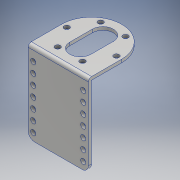
# Autodesk Inventor part: bepf_podwozie_lacznik_silnika
Saved by Autodesk Inventor 2017 (Build 210142000, 142)
## iProperties
Created: 2016-11-23
Part Number: bepf_podwozie_lacznik_silnika
Material: Aluminium 6061
Document SubType Name: Modeling
Designer: gagato
Density: 2.7 g/cm^3
Appearance: Aluminium — płaski
Mass: 14.4645 g
Surface Area: 63.668 cm^2
Volume: 5.35723 cm^3
Author: gagato
Autodesk Inventor part; units mm, degrees
ref_plane "YZ Plane" through (0, 0, 0) normal (1, 0, 0) x (0, 1, 0)
ref_plane "XZ Plane" through (0, 0, 0) normal (0, 1, 0) x (-1, 0, 0)
ref_plane "XY Plane" through (0, 0, 0) normal (0, 0, 1) x (1, 0, 0)
sketch "Szkic5" plane through (0, 0, 0) normal (0, 0, 1) x (1, 0, 0)
  line L0 (-18.8, 0) -> (18.8, 0)
  line L1 (0, 0) -> (0, 20.8) construction
  arc A0 (18.8, 20.8) -> (-18.8, 20.8) centre (0, 20.8) ccw
  line L2 (-18.8, 0) -> (-18.8, 20.8)
  line L3 (18.8, 0) -> (18.8, 20.8)
  circle A1 centre (0, 20.8) radius 15.5 construction
  line L4 (0, 27.8) -> (0, 13.8) construction
  line L5 (0, 27.8) -> (0, 13.8) construction
  line L6 (-6.6, 27.8) -> (-6.6, 13.8)
  line L7 (6.6, 13.8) -> (6.6, 27.8)
  arc A2 (6.6, 27.8) -> (-6.6, 27.8) centre (0, 27.8) ccw
  arc A3 (-6.6, 13.8) -> (6.6, 13.8) centre (0, 13.8) ccw
  point P0 (-15.5, 20.8)
  point P1 (0, 20.8)
  dimension "d35" = 31
  dimension "d26" = 37.6
  dimension "d27" = 20.8
  dimension "d28" = 37.6
  dimension "d46" = 14
  dimension "d47" = 13.2
  constraints: 18 end point, 6 point on circle, 4 tangent, 4 vertical, 3 centre point, 3 coincident, 3 midpoint, 2 equal length, 1 horizontal, 1 horizontal alignment, 2 other
  measures "d26" distance of L0.start L0.end
  measures "d27" distance of L1.end L1.start
  measures "d28" diameter of A0
  measures "d46" distance of L4.start L4.end
  measures "d47" diameter of A3
extrude "Wyciągnięcie proste4" add sketch "Szkic5" against normal blind 2 contours L2 A0 L3 L0 | A2 L7 A3 L6
sketch "Szkic6" plane through (18.8, 0, 0) normal (1, 0, 0) x (0, 0, -1)
  line L0 (2, 0) -> (2, 20.8) projected
  line L1 (2, 0) -> (51.2, 0)
  line L2 (51.2, 0) -> (51.2, 2)
  line L3 (51.2, 2) -> (2, 2)
  line L4 (2, 2) -> (2, 0)
  point P0 (0, 0)
  dimension "d31" = 49.2
  dimension "d32" = 2
  constraints: 8 end point, 2 parallel, 1 horizontal, 1 perpendicular
  measures "d31" distance of L3.end L2.end
  measures "d32" distance of L2.end L1.end
extrude "Wyciągnięcie proste5" add sketch "Szkic6" against normal up to surface (37.6 mm away)
hole "Otwór2" at (-15.5, 20.8, 0) direction (0, 0, -1) diameter 3.3 end through all
pattern_circular "Szyk kołowy2" count 6 over 360 about axis through (0, 20.8, 0) along (0, 0, -1) of "Otwór2"
extrude "Wyciągnięcie proste6" cut sketch "Szkic5" against normal through all contours A2 L7 A3 L6
sketch "Szkic7" plane through (18.8, 2, -2) normal (0, 1, 0) x (1, 0, 0)
  line L0 (-18.8, -2) -> (-18.8, 44.5) construction
  line L1 (-34.4, 44.5) -> (-3.2, 44.5) construction
  dimension "d50" = 31.2
  dimension "d51" = 46.5
  constraints: 4 end point, 1 coincident, 1 horizontal, 1 midpoint, 1 vertical
  measures "d50" distance of L1.start L1.end
  measures "d51" distance of L0.start L0.end
hole "Otwór3" at (-15.6, 2, -46.5) direction (0, -1, 0) diameter 3.2 end through all
pattern_linear "Szyk prostokątny1" count 7 spacing 6.4 along (0, 0, 1) of "Otwór3"
mirror "Odbij1" about plane through (0, 0, 0) normal (1, 0, 0) of "Otwór3", "Szyk prostokątny1"
fillet "Zaokrąglenie1" radius 4 2 edges at (18.8, 1, -51.2) (-18.8, 1, -51.2)
fillet "Zaokrąglenie2" radius 2 1 edges at (0, 0, 0)
